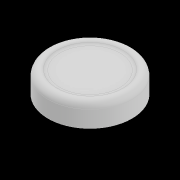
# Autodesk Inventor part: Boton Tapa
Saved by Autodesk Inventor 2020 (Build 240168000, 168)
## iProperties
Created: 2022-02-20
Part Number: Boton Tapa
Material: Genérico
Document SubType Name: Modeling
Designer: Alférez
Density: 1 g/cm^3
Appearance: Valor por defecto
Author: Alférez
Autodesk Inventor part; units mm, degrees
ref_plane "YZ Plane" through (0, 0, 0) normal (1, 0, 0) x (0, 1, 0)
ref_plane "XZ Plane" through (0, 0, 0) normal (0, 1, 0) x (-1, 0, 0)
ref_plane "XY Plane" through (0, 0, 0) normal (0, 0, 1) x (1, 0, 0)
sketch "Boceto1" plane through (0, 0, 0) normal (0, 1, 0) x (-1, 0, 0)
  circle A0 centre (0, 0) radius 7
  dimension "d0" = 14
  constraints: 1 centre point, 1 coincident
  measures "d0" diameter of A0
extrude "Extrusión1" add sketch "Boceto1" along normal blind 2
sketch "Boceto2" plane through (0, 0, 0) normal (0, -1, 0) x (1, 0, 0)
  circle A0 centre (0, 0) radius 5.625
  circle A1 centre (0, 0) radius 7
  dimension "d3" = 11.25
  dimension "d4" = 14
  constraints: 2 centre point, 2 coincident
  measures "d3" diameter of A0
  measures "d4" diameter of A1
extrude "Extrusión2" add sketch "Boceto2" along normal blind 2.5
sketch "Boceto3" plane through (0, 0, 0) normal (0, -1, 0) x (1, 0, 0)
  line L0 (0, 0) -> (3, 0)
  line L1 (3, 0) -> (3, -1.5)
  line L2 (3, -1.5) -> (1.5, -1.5)
  line L3 (1.5, -1.5) -> (1.5, -3)
  line L4 (1.5, -3) -> (-1.5, -3)
  line L5 (-1.5, -3) -> (-1.5, -1.5)
  line L6 (-1.5, -1.5) -> (-3, -1.5)
  line L7 (-3, -1.5) -> (-3, 1.5)
  line L8 (-3, 1.5) -> (-1.5, 1.5)
  line L9 (-1.5, 1.5) -> (-1.5, 3)
  line L10 (-1.5, 3) -> (1.5, 3)
  line L11 (1.5, 3) -> (1.5, 1.5)
  line L12 (1.5, 1.5) -> (3, 1.5)
  line L13 (3, 1.5) -> (3, 0)
  line L14 (-1.5, 1.5) -> (1.5, 1.5)
  line L15 (1.5, 1.5) -> (1.5, -1.5)
  line L16 (1.5, -1.5) -> (-1.5, -1.5)
  line L17 (-1.5, -1.5) -> (-1.5, 1.5)
  line L18 (-1.5, 1.5) -> (1.5, 1.5)
  line L19 (1.5, 1.5) -> (1.5, -1.5)
  line L20 (1.5, -1.5) -> (-1.5, -1.5)
  line L21 (-1.5, -1.5) -> (-1.5, 1.5)
  dimension "d7" = 3
  dimension "d8" = 1.5
  dimension "d9" = 1.5
  dimension "d10" = 1.5
  dimension "d11" = 3
  dimension "d12" = 1.5
  dimension "d13" = 1.5
  dimension "d14" = 3
  dimension "d15" = 1.5
  dimension "d16" = 1.5
  dimension "d17" = 3
  dimension "d18" = 1.5
  dimension "d19" = 1.5
  constraints: 44 end point, 8 perpendicular, 7 point on line, 4 parallel, 3 horizontal
  measures "d7" distance of L0.start L0.end
  measures "d8" distance of L0.end L1.end
  measures "d9" distance of L1.end L2.end
  measures "d10" distance of L2.end L3.end
  measures "d11" distance of L3.end L4.end
  measures "d12" distance of L4.end L5.end
  measures "d13" distance of L5.end L6.end
  measures "d14" distance of L6.end L7.end
  measures "d15" distance of L7.end L8.end
  measures "d16" distance of L8.end L9.end
  measures "d17" distance of L9.end L10.end
  measures "d18" distance of L10.end L11.end
  measures "d19" distance of L11.end L12.end
extrude "Extrusión3" add sketch "Boceto3" along normal blind 5 contours L15 L16 L17 L14
sketch "Boceto8" plane through (0, 2, 0) normal (0, 1, 0) x (1, 0, 0)
  circle A0 centre (0, 0) radius 6
  dimension "d55" = 12
  constraints: 1 centre point, 1 coincident
  measures "d55" diameter of A0
extrude "Extrusión6" cut sketch "Boceto8" against normal blind 1
fillet "Empalme2" radius 1 3 edges at (-6, 1, 0) (-6, 2, 0) (7, 2, 0)
fillet "Empalme5" radius 1 4 edges at (1.5, -2.5, 1.5) (-1.5, -2.5, 1.5) (1.5, -2.5, -1.5) (-1.5, -2.5, -1.5)
